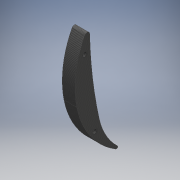
# Autodesk Inventor part: styro_50_main_center
Saved by Autodesk Inventor 2018.2 (Build 222227000, 227)
## iProperties
Created: 2017-12-11
Part Number: styro_50_main_center
Material: ポリスチレン、耐衝撃性
Document SubType Name: Modeling
Designer: kuwano
Density: 1.022 g/cm^3
Appearance: カーボンファイバー
Mass: 1183.2 g
Surface Area: 1012.81 cm^2
Volume: 1157.73 cm^3
Author: kuwano
Autodesk Inventor part; units mm, degrees
ref_plane "YZ Plane" through (0, 0, 0) normal (1, 0, 0) x (0, 1, 0)
ref_plane "XZ Plane" through (0, 0, 0) normal (0, 1, 0) x (-1, 0, 0)
ref_plane "XY Plane" through (0, 0, 0) normal (0, 0, 1) x (1, 0, 0)
sketch "スケッチ1" plane through (0, 0, 0) normal (1, 0, 0) x (0, 1, 0)
  line L0 (0, 0) -> (147.3717, -500)
  arc A0 (0, 0) -> (37.8967, -343.7392) centre (1577.8776, 0) ccw
  arc A1 (37.8967, -343.7392) -> (147.3717, -500) centre (281.8923, -289.2769) ccw
  arc A2 (0, 0) -> (-50, -259.8835) centre (293.1864, -191.1589) ccw
  arc A3 (-50, -259.8835) -> (147.3717, -500) centre (273.5758, -195.086) ccw
  line L1 (0, -630.6128) -> (0, 110.8282) projected
  point P0 (35.1596, -247.5153)
  dimension "d1" = 500
  dimension "d2" = 250
  dimension "d3" = 1577.8776
  dimension "d4" = 250
  dimension "d6" = 350
  dimension "d21" = 330
  dimension "d26" = 50
  constraints: 8 point on circle, 4 centre point, 3 tangent, 2 end point, 1 coincident
  measures "d1" vertical distance of L0.end L0.start
  measures "d2" distance of point (35.16, -247.515) L0.start
  measures "d3" radius of A0
  measures "d4" radius of A1
  measures "d6" radius of A2
  measures "d21" radius of A3
  measures "d26" horizontal distance of A2.end point (0, 0)
extrude "押し出し1" add sketch "スケッチ1" along normal mid plane 50 contours L1 A3 A2 | A0 A1 A3 L1
fillet "フィレット1" radius 10 1 edges at (0, 0, 0)
fillet "フィレット1" radius 5 1 edges at (0, 147.3717, -500)
sketch "スケッチ2" plane through (25, 0, 0) normal (1, 0, 0) x (0, 0, -1)
  circle A0 centre (96.4602, -19.5814) radius 7.5
  circle A1 centre (376.4602, 20.4186) radius 7.5
  arc A2 (36.2306, 0.416) -> (31.9103, -18.4863) centre (36.4602, -9.5814) ccw projected
  point P0 (0, 0)
  dimension "d11" = 15
  dimension "d12" = 15
  dimension "d13" = 280
  dimension "d16" = 40
  dimension "d24" = 60
  dimension "d25" = 10
  constraints: 2 centre point
  measures "d11" diameter of A1
  measures "d12" diameter of A0
  measures "d13" horizontal distance of A1.centre A0.centre
  measures "d16" vertical distance of A1.centre A0.centre
  measures "d24" horizontal distance of A2.centre A0.centre
  measures "d25" vertical distance of A2.centre A0.centre
extrude "押し出し2" cut sketch "スケッチ2" against normal through all
